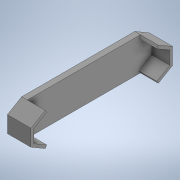
# Autodesk Inventor part: HexWheelGuard
Saved by Autodesk Inventor 2020 (Build 240168000, 168)
## iProperties
Created: 2023-12-19
Part Number: HexWheelGuard
Material: H TPU
Document SubType Name: Modeling
Designer: smz3rm
Density: 0.941117 g/cm^3
Appearance: Generic(1)
Mass: 33.4085 g
Surface Area: 159.906 cm^2
Volume: 35.4988 cm^3
Author: smz3rm
Autodesk Inventor part; units mm, degrees
ref_plane "YZ Plane" through (0, 0, 0) normal (1, 0, 0) x (0, 1, 0)
ref_plane "XZ Plane" through (0, 0, 0) normal (0, 1, 0) x (-1, 0, 0)
ref_plane "XY Plane" through (0, 0, 0) normal (0, 0, 1) x (1, 0, 0)
sketch "Sketch1" plane through (0, 0, 0) normal (1, 0, 0) x (0, 1, 0)
  line L0 (-17.5, 75) -> (17.5, 75)
  line L1 (17.5, 75) -> (17.5, -75)
  line L2 (17.5, -75) -> (-17.5, -75)
  line L3 (-17.5, -75) -> (-17.5, 75)
  line L4 (-17.5, 75) -> (17.5, -75) construction
  line L5 (17.5, 75) -> (-17.5, -75) construction
  line L6 (17.5, 64.8964) -> (17.5, 43.9858)
  line L7 (-17.5, 43.9858) -> (-17.5, 64.1931)
  line L8 (-24.5, 0) -> (24.5, 0) projected
  line L9 (0, -105) -> (0, 105) projected
  line L10 (-17.5, -59.8446) -> (-8.75, -44.6891)
  line L11 (-8.75, -44.6891) -> (8.75, -44.6891)
  line L12 (8.75, -44.6891) -> (17.5, -59.8446)
  line L13 (17.5, -59.8446) -> (8.75, -75)
  line L14 (8.75, -75) -> (-8.75, -75)
  line L15 (-8.75, -75) -> (-17.5, -59.8446)
  line L16 (17.5, 59.8446) -> (8.75, 75)
  line L17 (-8.75, 75) -> (-17.5, 59.8446)
  point P0 (0, 0)
  point P1 (0, -59.8446)
  point P2 (-8.75, -75)
  dimension "d0" = 35
  dimension "d1" = 150
  constraints: 32 end point, 4 symmetric about line, 3 collinear, 2 midpoint, 2 parallel, 2 point on line, 1 horizontal, 1 perpendicular, 13 other
  measures "d0" distance of L1.end L2.end
  measures "d1" distance of L0.end L1.end
extrude "Extrusion1" add sketch "Sketch1" along normal blind 6 contours L0 L9 L8 L3 L17 | L0 L16 L1 L8 L9 | L9 L11 L10 L3 L8 | L8 L1 L12 L11 L9 | L11 L12 L13 L2 L9 | L9 L2 L15 L10 L11
sketch "Sketch2" plane through (6, 0, 0) normal (1, 0, 0) x (0, 0, -1)
  line L0 (-59.8446, 17.5) -> (-75, 8.75) projected
  line L1 (-75, 8.75) -> (-75, -8.75) projected
  line L2 (-75, -8.75) -> (-59.8446, -17.5) projected
  line L3 (-58.3446, 14.9019) -> (-72, 7.0179)
  line L4 (-72, 7.0179) -> (-72, -7.0179)
  line L5 (-72, -7.0179) -> (-58.3446, -14.9019)
  line L6 (-58.3446, 14.9019) -> (-59.8446, 17.5)
  line L7 (-58.3446, -14.9019) -> (-59.8446, -17.5)
  line L8 (75, 8.75) -> (59.8446, 17.5) projected
  line L9 (59.8446, -17.5) -> (75, -8.75) projected
  line L10 (75, -8.75) -> (75, 8.75) projected
  line L11 (58.3446, 14.9019) -> (72, 7.0179)
  line L12 (72, 7.0179) -> (72, -7.0179)
  line L13 (72, -7.0179) -> (58.3446, -14.9019)
  line L14 (59.8446, 17.5) -> (-59.8446, 17.5) projected
  line L15 (58.3446, 14.9019) -> (59.8446, 17.5)
  line L16 (58.3446, -14.9019) -> (59.8446, -17.5)
  point P0 (0, 0)
  dimension "d4" = 3
  dimension "d7" = 3
  constraints: 20 end point, 4 perpendicular, 4 other
  measures "d4" distance between parallel lines of L0 L3
  measures "d7" distance between parallel lines of L8 L11
extrude "Extrusion2" add sketch "Sketch2" along normal blind 19
equation "\"d0\" = BodyHeight"
equation "\"d1\" = BodyLength"
equation "\"d2\" = SideThickness"
equation "\"d5\" = WheelSlotWidth"
equation "\"BodyHeight\" = 35"
equation "\"BodyLength\" = 150"
equation "\"SideThickness\" = 6"
equation "\"WheelSlotWidth\" = 19"
body "Solid1"
